Autodesk Fusion 360 part; units mm, degrees
note: some values were not read from the file. Set by a fixed rule: which face or edge a step refers to.
(part 2 of 2)
  line L360 (0, -123.825) -> (309.5625, -123.825)
  line L361 (0, 0) -> (309.5625, 0)
  line L362 (0, -123.825) -> (0, 0)
  line L363 (309.5625, -123.825) -> (309.5625, 0)
extrude "Extrude1" add sketch "plate-2026-03-22T13_27_17.077Z" along normal blind 1.5 makes body 1
extrude "Extrude2" add 1 faces at (0, -82.55, 0.5) along direction (-1, 0, 0) blind 2 separate body on bodies 1 makes body 2
extrude "Extrude3" add 2 faces at (103.1875, -123.825, 0.5) (-0.6667, -123.825, 0.5) along direction (0, -1, 0) blind 1 separate body on bodies 1 2 makes body 3
extrude "Extrude4" add 2 faces at (309.5625, -82.55, 0.5) (309.5625, -124.1583, 0.5) along direction (1, 0, 0) blind 1 separate body on bodies 1 3 makes body 4
extrude "Extrude5" add 1 faces at (310.5625, -41.275, 1) along direction (1, 0, 0) blind 1 on bodies 4 bodies 4
extrude "Extrude6" add 3 faces at (310.2292, 0, 0.5) (103.1875, 0, 0.5) (-0.6667, 0, 0.5) along direction (0, 1, 0) blind 12 separate body on bodies 1 2 4 makes body 5
combine "Combine1" operation add target body 5 tool bodies 2 3 4
extrude "Extrude7" add 1 faces at (311.5625, -79.2167, 0.5) along direction (1, 0, 0) blind 2 separate body on bodies 5 makes body 6
extrude "Extrude8" add 2 faces at (102.5208, -124.825, 0.5) (312.2292, -124.825, 0.5) along direction (0, -1, 0) blind 2 separate body on bodies 5 6 makes body 7
extrude "Extrude9" add 2 faces at (-2, -33.6083, 1) (-2, -125.4917, 0.5) along direction (-1, 0, 0) blind 2 separate body on bodies 5 7 makes body 8
extrude "Extrude10" add 3 faces at (207.0417, 12, 1) (-2.6667, 12, 0.5) (312.2292, 12, 0.5) along direction (0, 1, 0) blind 2 separate body on bodies 5 6 8 makes body 9
extrude "Extrude11" add 8 faces at (-2.6667, 12.6667, 0) (102.5208, 12.6667, 0) (312.2292, 12.6667, 0) (312.2292, -33.6083, 0) (-2.6667, -125.4917, 0) (-2.6667, -79.2167, 0) (207.0417, -125.4917, 0) (312.2292, -125.4917, 0) along direction (0, 0, -1) blind 20 on bodies 6 7 8 9 bodies 5 9 6 7 8
sketch "Sketch2" plane through (0, 0, -20) normal (0, 0, -1) x (1, 0, 0)
  line L0 (313.5625, 126.825) -> (-4, 126.825)
  line L1 (-4, 126.825) -> (-4, -14)
  line L2 (-4, -14) -> (313.5625, -14)
  line L3 (313.5625, -14) -> (313.5625, 126.825)
  line L4 (-2, 124.825) -> (311.5625, 124.825)
  line L5 (311.5625, 124.825) -> (311.5625, -12)
  line L6 (311.5625, -12) -> (-2, -12)
  line L7 (-2, -12) -> (-2, 124.825)
  line L8 (-4, 126.825) -> (313.5625, 126.825)
  line L9 (313.5625, 126.825) -> (313.5625, -14)
  line L10 (313.5625, -14) -> (-4, -14)
  line L11 (-4, -14) -> (-4, 126.825)
  constraint horizontal L8
  constraint vertical L9
  constraint horizontal L10
  constraint vertical L11
  constraint coincident L2.end L3.start
  constraint coincident L0.end L1.start
extrude "Extrude12" add sketch "Sketch2" against normal blind 3 contours L4 L5 L6 L7 bodies 5
extrude "Extrude13" cut 1 faces at (101.8542, -79.8833, -20) along direction (0, 0, 1) blind 4 on bodies 5 bodies 5
sketch "Sketch3" plane through (0, 0, -16) normal (0, 0, -1) x (1, 0, 0)
  line L0 (-2, 124.825) -> (311.5625, 124.825)
  line L1 (311.5625, 124.825) -> (311.5625, -12)
  line L2 (311.5625, -12) -> (-2, -12)
  line L3 (-2, -12) -> (-2, 124.825)
  line L4 (313.5625, 126.825) -> (-4, 126.825)
  line L5 (-4, 126.825) -> (-4, -14)
  line L6 (-4, -14) -> (313.5625, -14)
  line L7 (313.5625, -14) -> (313.5625, 126.825)
extrude "Extrude14" add sketch "Sketch3" against normal blind 3 contours L0 L1 L2 L3 bodies 5
